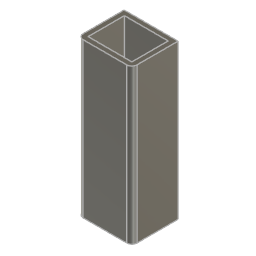
battery_holder (Autodesk Fusion 360 design; units mm, degrees)
Autodesk Fusion 360 part; units mm, degrees
sketch "Sketch1" plane through (0, 0, 0) normal (0, 0, 1) x (1, 0, 0)
  line L0 (0, 0) -> (17, 0)
  line L1 (17, 0) -> (17, 14.1)
  line L2 (17, 14.1) -> (0, 14.1)
  line L3 (0, 14.1) -> (0, 0)
  line L4 (-2, -2) -> (19, -2)
  line L5 (19, -2) -> (19, 16)
  line L6 (19, 16) -> (-2, 16)
  line L7 (-2, 16) -> (-2, -2)
  dimension "d1" = 17
  dimension "d2" = 14.1
  constraint horizontal L0
  constraint vertical L1
  constraint horizontal L2
  constraint vertical L3
  constraint coincident L0.start L3.end
  constraint horizontal L4
  constraint vertical L5
  constraint horizontal L6
  constraint vertical L7
  measures "d1" distance of L0.start L0.end
  measures "d2" distance of L0.start L2.end
extrude "Extrude1" add sketch "Sketch1" along normal blind 60
fillet "Fillet1" radius 2 2 edges at (-2, -2, 30) (19, -2, 30)
